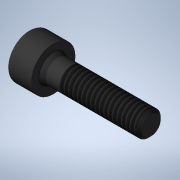
# Autodesk Inventor part: Slotted head cap screw ISO 4762 - M2.5x10
Saved by Autodesk Inventor 2021 (Build 250183000, 183)
## iProperties
Created: 2024-12-08
Part Number: Slotted head cap screw ISO 4762 - M2.5x10
Material: Generic
Catalog Web Link: www.cadenas.de
Description: ISO 4762-Hexagon socket head cap screw
Vendor: MISUMI
Document SubType Name: Modeling
Designer: psAdmin
Manufacturer: MISUMI
Mass: 0.0825143 g
Surface Area: 1.52973 cm^2
Volume: 0.0825143 cm^3
Density: 1 g/cm^3
Appearance: PSOLRGB-175-175-175
Category: PARTsolutions
Company: MISUMI
Title: Slotted head cap screw ISO 4762 - M2.5x10
Author: Cadenas PARTsolutions
Comments: Hexagon socket head cap screw
PSOL_IDENT_0: {$CADENAS_DATA/23d-libs/misumi/metric/accessories/din_en_iso_4762.prj},225 {VTYP=3D},{NB=Slotted hea
PSOL_IDENT_1: d cap screw ISO 4762 - M2.5x10},{LINA=Slotted head cap screw ISO 4762 - M2.5x10},{NN=ISO 4762},{DATE=
PSOL_IDENT_2: 29.11.2024 04:47:06},{GEOMDATE=05.09.2023 10:22:53},{VERSION=},{LINEID=230},{WBVAR=},{WBNUMERIC=}  {
PSOL_IDENT_3: NB=Zylinderschraube ISO 4762 - M2.5x10},{LINA=Zylinderschraube ISO 4762 - M2.5x10},{KT=DUMMY},{IDNR=
PSOL_IDENT_4: },{D=2.500},{D3=1.948},{P=0.450},{L=10.000},{S=2.000},{DK=4.500},{DA=3.100},{DS=2.500},{E=2.300},{K=
PSOL_IDENT_5: 2.500},{R=0.100},{T=1.100},{V=0.250},{DW=4.180},{W=0.850},{HM=10.000},{LF=0.510},{LG=1.350},{FORM=1.
PSOL_IDENT_6: 000},{NENN=M2.5x10}
NB: Slotted head cap screw ISO 4762 - M2.5x10
NN: ISO 4762
NT: Hexagon socket head cap screw
NBSYN: Slotted head cap screw ISO 4762 - $NENN.
LINA: Slotted head cap screw ISO 4762 - M2.5x10
CATALOG: Misumi
ROWDESC: M2.5x10
D: 2.5
D3: 1.948
P: 0.45
L: 10
S: 2
DK: 4.5
DA: 3.1
DS: 2.5
E: 2.3
K: 2.5
R: 0.1
T: 1.1
V: 0.25
DW: 4.18
W: 0.85
HM: 10
LF: 0.51
LG: 1.35
FORM: 1
SUPPLIER: MISUMI
ARTICLENO: Slotted head cap screw ISO 4762 - M2.5x10
BOMINFO: Slotted head cap screw ISO 4762 - M2.5x10
CREATOR: CADENAS GmbH
Autodesk Inventor part; units mm, degrees
sketch "Sketch_1" plane through (0, 0, 0) normal (0, 1, 0) x (-1, 0, 0)
  line L0 (-10, 0) -> (5.5, 0)
  line L1 (0.2726, 0) -> (0.85, -1)
  line L2 (0.85, -1) -> (2.35, -1)
  line L3 (2.35, -1) -> (2.5, -1.15)
  line L4 (2.5, -1.15) -> (2.5, -2)
  arc A0 (2.25, -2.25) -> (2.5, -2) centre (2.25, -2) ccw
  line L5 (2.25, -2.25) -> (0, -2.25)
  line L6 (0, -2.25) -> (0, -1.55)
  arc A1 (0, -1.55) -> (-0.0562, -1.4601) centre (-0.1, -1.55) ccw
  line L7 (-0.0562, -1.4601) -> (-0.4662, -1.2601)
  arc A2 (-0.4662, -1.2601) -> (-0.51, -1.25) centre (-0.51, -1.35) ccw
  line L8 (-0.51, -1.25) -> (-9.724, -1.25)
  line L9 (-9.724, -1.25) -> (-10, -0.974)
  line L10 (-10, -0.974) -> (-10, 0)
  line L11 (-10, 0) -> (0.2726, 0)
  constraints: 24 end point, 6 point on circle, 3 centre point
revolve "Revolution1" add sketch "Sketch_1" angle 360 about axis through (10, 0, 0) along (1, 0, 0)
thread "Thread1" size "M2.5x0.45" class "6g" standard "ISO Metric profile" length 7.864
sketch "Skizze_1" plane through (-0.85, 0, 0) normal (1, 0, 0) x (0, 0, -1)
  line L0 (-1, -0.5774) -> (0, -1.1547)
  line L1 (0, -1.1547) -> (1, -0.5774)
  line L2 (1, -0.5774) -> (1, 0.5774)
  line L3 (1, 0.5774) -> (0, 1.1547)
  line L4 (0, 1.1547) -> (-1, 0.5774)
  line L5 (-1, 0.5774) -> (-1, -0.5774)
  constraints: 12 end point
extrude "Extrusion1" cut sketch "Skizze_1" against normal blind 2.2
ref_plane "IP1_XY" through (0, 0, 0) normal (1, 0, 0) x (0, 0, -1)
ref_plane "IP1_YZ" through (0, 0, 0) normal (0, 0, -1) x (0, 1, 0)
ref_plane "IP1_ZX" through (0, 0, 0) normal (0, 1, 0) x (1, 0, 0)
ref_plane "IP2_XY" through (-2.5, 0, 0) normal (1, 0, 0) x (0, 0, -1)
ref_plane "IP2_YZ" through (-2.5, 0, 0) normal (0, 0, -1) x (0, 1, 0)
ref_plane "IP2_ZX" through (-2.5, 0, 0) normal (0, 1, 0) x (1, 0, 0)
ref_plane "IP3_XY" through (10, 0, 0) normal (1, 0, 0) x (0, 0, -1)
ref_plane "IP3_YZ" through (10, 0, 0) normal (0, 0, -1) x (0, 1, 0)
ref_plane "IP3_ZX" through (10, 0, 0) normal (0, 1, 0) x (1, 0, 0)
ref_plane "IP4_XY" through (0, 0, 0) normal (1, 0, 0) x (0, 0, -1)
ref_plane "IP4_YZ" through (0, 0, 0) normal (0, 0, -1) x (0, 1, 0)
ref_plane "IP4_ZX" through (0, 0, 0) normal (0, 1, 0) x (1, 0, 0)
body "Solid1"
